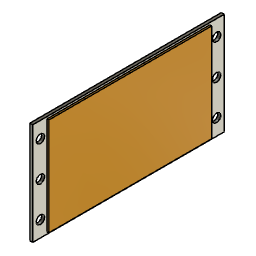
Reflektor v12 (Autodesk Fusion 360 archive; units mm, degrees)
design "LED"
Autodesk Fusion 360 part; units mm, degrees
sketch "Sketch1" plane through (0, 0, 0) normal (1, 0, 0) x (0, 1, 0) in component "Led"
  line L0 (47, 25) -> (-47, 25)
  line L1 (-47, 25) -> (-47, -25)
  line L2 (-47, -25) -> (47, -25)
  line L3 (47, -25) -> (47, 25)
  line L4 (47, 25) -> (-47, -25) construction
  line L5 (-47, 25) -> (47, -25) construction
  line L6 (40, -24) -> (-40, -24)
  line L7 (-40, -24) -> (-40, 24)
  line L8 (-40, 24) -> (40, 24)
  line L9 (40, 24) -> (40, -24)
  line L10 (40, -24) -> (-40, 24) construction
  line L11 (-40, -24) -> (40, 24) construction
  circle A0 centre (43.25, 0) radius 2.05
  line L12 (43.25, 0) -> (43.25, 17.2) construction
  line L13 (43.25, 0) -> (43.25, -17.2) construction
  circle A1 centre (43.25, 17.2) radius 2.05
  circle A2 centre (43.25, -17.2) radius 2.05
  line L14 (0, 25) -> (0, -25) construction
  circle A3 centre (-43.25, 17.2) radius 2.05
  circle A4 centre (-43.25, 0) radius 2.05
  circle A5 centre (-43.25, -17.2) radius 2.05
  line L15 (39.5, 24) -> (-39.5, 24) construction
  line L16 (-39.5, 24) -> (-39.5, -24) construction
  line L17 (-39.5, -24) -> (39.5, -24) construction
  line L18 (39.5, -24) -> (39.5, 24) construction
  line L19 (39.5, 24) -> (-39.5, -24) construction
  line L20 (-39.5, 24) -> (39.5, -24) construction
  line L21 (39.5, 0) -> (47, 0) construction
  dimension "d9" = 94
  dimension "d10" = 50
  dimension "d11" = 80
  dimension "d12" = 48
  dimension "d13" = 4.1
  dimension "d14" = 17.2
  dimension "d15" = 17.2
  dimension "d16" = 4.1
  dimension "d17" = 4.1
  dimension "d24" = 79
  dimension "d25" = 48
  constraint horizontal L0
  constraint perpendicular L0 L1
  constraint parallel L0 L2
  constraint parallel L1 L3
  constraint coincident L4 origin
  constraint coincident L5 origin
  constraint horizontal L6
  constraint perpendicular L6 L7
  constraint parallel L6 L8
  constraint parallel L7 L9
  constraint coincident L10 origin
  constraint coincident L11 origin
  constraint coincident A0.centre L12.start
  constraint perpendicular L2 L13
  constraint coincident L12.end A1.centre
  constraint coincident L13.end A2.centre
  constraint midpoint L0 L14.start
  constraint midpoint L2 L14.end
  constraint symmetric A0 L14 A4
  constraint symmetric A1 L14 A3
  constraint symmetric A2 L14 A5
  constraint horizontal L15
  constraint perpendicular L15 L16
  constraint parallel L15 L17
  constraint parallel L16 L18
  constraint coincident L19 origin
  constraint coincident L20 origin
  constraint midpoint L18 L21.start
  constraint midpoint L3 L21.end
  constraint midpoint A0.centre L21
  constraint parallel L12 L13
  measures "d9" distance of L1.end L2.end
  measures "d10" distance of L0.end L1.end
  measures "d11" distance of L7.end L8.end
  measures "d12" distance of L6.end L7.end
  measures "d13" diameter of A0
  measures "d14" distance of A0.centre L12.end
  measures "d15" distance of A0.centre L13.end
  measures "d16" diameter of A1
  measures "d17" diameter of A2
  measures "d24" distance of L16.end L17.end
  measures "d25" distance of L15.end L16.end
extrude "Extrude1" add sketch "Sketch1" along normal blind 1.4 contours L0 L1 L2 L3 | L6 L7 L8 L9 in component "Led"
extrude "Extrude2" add sketch "Sketch1" along normal blind 2.3 contours L6 L7 L8 L9 in component "Led"
component "Led" placed x (1, 0, 0) y (0, 1, 0) z (0, 0, 1) at (1.4097, 0.3286, -4.1948)
equation "Širina = 94 mm"
equation "mala_širina = 80 mm"
equation "višina = 50 mm"
equation "mala_višina = višina - 2 mm"
equation "razdalja_med_luknjami = 17.2 mm"
equation "fi = 4.1 mm"
equation "debelina = 1.4 mm"
equation "velika_debelina = 2.3 mm"
equation "d9 = Širina"
equation "d10 = višina"
equation "d11 = mala_širina"
equation "d12 = mala_višina"
equation "d13 = fi"
equation "d14 = razdalja_med_luknjami"
equation "d15 = razdalja_med_luknjami"
equation "d16 = fi"
equation "d17 = fi"
equation "d18 = debelina"
equation "d20 = velika_debelina"
equation "namišljena_mala_višina = 79 mm"
equation "d24 = namišljena_mala_višina"
equation "d25 = mala_višina"

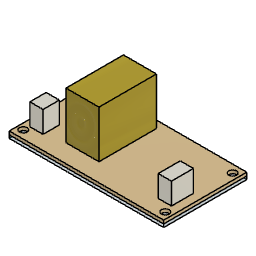
design "Napajalnik 12v 2a"
Autodesk Fusion 360 part; units mm, degrees
sketch "Sketch1" plane through (0, 0, 0) normal (0, 0, 1) x (1, 0, 0)
  line L0 (35.115, -18.89) -> (-35.115, -18.89)
  line L1 (-35.115, -18.89) -> (-35.115, 18.89)
  line L2 (-35.115, 18.89) -> (35.115, 18.89)
  line L3 (35.115, 18.89) -> (35.115, -18.89)
  line L4 (35.115, -18.89) -> (-35.115, 18.89) construction
  line L5 (-35.115, -18.89) -> (35.115, 18.89) construction
  circle A0 centre (-32.37, 15.345) radius 1.745
  circle A1 centre (32.24, 15.345) radius 1.745
  circle A2 centre (-32.37, -15.245) radius 1.745
  circle A3 centre (32.24, -15.245) radius 1.745
  line L6 (31.315, -1.56) -> (25.315, -1.56)
  line L7 (25.315, -1.56) -> (25.315, -11.56)
  line L8 (25.315, -11.56) -> (31.315, -11.56)
  line L9 (31.315, -11.56) -> (31.315, -1.56)
  line L10 (35.115, 15.345) -> (33.985, 15.345) construction
  line L11 (33.985, -15.245) -> (35.115, -15.245) construction
  line L12 (32.24, 18.89) -> (32.24, 17.09) construction
  line L13 (32.24, -16.99) -> (32.24, -18.89) construction
  line L14 (31.315, -11.56) -> (35.115, -11.56) construction
  line L15 (31.315, -11.56) -> (31.315, -18.89) construction
  line L16 (-32.37, -16.99) -> (-32.37, -18.89) construction
  line L17 (-34.115, -15.245) -> (-35.115, -15.245) construction
  line L18 (-32.37, 17.09) -> (-32.37, 18.89) construction
  line L19 (-34.115, 15.345) -> (-35.115, 15.345) construction
  line L20 (-32.115, -5.12) -> (-26.115, -5.12)
  line L21 (-26.115, -5.12) -> (-26.115, -12.52)
  line L22 (-26.115, -12.52) -> (-32.115, -12.52)
  line L23 (-32.115, -12.52) -> (-32.115, -5.12)
  line L24 (-32.115, -12.52) -> (-32.115, -18.89) construction
  line L25 (-32.115, -12.52) -> (-35.115, -12.52) construction
  line L26 (-17.615, 15.55) -> (-2.615, 15.55)
  line L27 (-2.615, 15.55) -> (-2.615, -10.59)
  line L28 (-2.615, -10.59) -> (-17.615, -10.59)
  line L29 (-17.615, -10.59) -> (-17.615, 15.55)
  line L30 (-10.115, -10.59) -> (-10.115, -18.89) construction
  line L31 (-17.615, 15.55) -> (-35.115, 15.345) construction
  dimension "d1" = 70.23
  dimension "d2" = 37.78
  dimension "d3" = 3.49
  dimension "d4" = 3.49
  dimension "d5" = 3.49
  dimension "d6" = 3.49
  dimension "d7" = 6
  dimension "d8" = 10
  dimension "d9" = 1.13
  dimension "d10" = 1.13
  dimension "d11" = 1.8
  dimension "d12" = 1.9
  dimension "d13" = 3.8
  dimension "d14" = 7.33
  dimension "d15" = 1
  dimension "d16" = 1
  dimension "d17" = 6
  dimension "d18" = 7.4
  dimension "d19" = 6.37
  dimension "d20" = 3
  dimension "d21" = 15
  dimension "d22" = 26.14
  dimension "d23" = 8.3
  dimension "d24" = 17.5
  constraint horizontal L0
  constraint perpendicular L0 L1
  constraint parallel L0 L2
  constraint parallel L1 L3
  constraint coincident L4 origin
  constraint coincident L5 origin
  constraint horizontal L6
  constraint vertical L7
  constraint horizontal L8
  constraint vertical L9
  constraint coincident L3 L10.start
  constraint coincident A1 L10.end
  constraint perpendicular L3 L10
  constraint coincident A1.centre L10
  constraint coincident A3 L11.start
  constraint coincident L3 L11.end
  constraint perpendicular L3 L11
  constraint coincident A3.centre L11
  constraint coincident L2 L12.start
  constraint coincident A1 L12.end
  constraint perpendicular L2 L12
  constraint coincident A1.centre L12
  constraint coincident A3 L13.start
  constraint coincident L0 L13.end
  constraint perpendicular L0 L13
  constraint coincident A3.centre L13
  constraint coincident L3 L14.end
  constraint perpendicular L3 L14
  constraint coincident L0 L15.end
  constraint perpendicular L0 L15
  constraint coincident A2 L16.start
  constraint coincident L0 L16.end
  constraint perpendicular L0 L16
  constraint coincident A2.centre L16
  constraint coincident A2 L17.start
  constraint coincident L1 L17.end
  constraint perpendicular L1 L17
  constraint coincident A2.centre L17
  constraint coincident A0 L18.start
  constraint coincident L2 L18.end
  constraint perpendicular L2 L18
  constraint coincident A0 L19.start
  constraint coincident L1 L19.end
  constraint perpendicular L1 L19
  constraint coincident A0.centre L18
  constraint coincident A0.centre L19
  constraint equal L12 L18
  constraint equal L13 L16
  constraint horizontal L20
  constraint vertical L21
  constraint horizontal L22
  constraint vertical L23
  constraint coincident L0 L24.end
  constraint perpendicular L0 L24
  constraint coincident L1 L25.end
  constraint perpendicular L1 L25
  constraint horizontal L26
  constraint vertical L27
  constraint horizontal L28
  constraint vertical L29
  constraint midpoint L28 L30.start
  constraint coincident L0 L30.end
  constraint perpendicular L0 L30
  measures "d1" distance of L1.end L2.end
  measures "d2" distance of L0.end L1.end
  measures "d3" diameter of A0
  measures "d4" diameter of A1
  measures "d5" diameter of A2
  measures "d6" diameter of A3
  measures "d7" distance of L6.start L6.end
  measures "d8" distance of L6.start L8.end
  measures "d9" distance of L10.start L10.end
  measures "d10" distance of L11.start L11.end
  measures "d11" distance of L12.start L12.end
  measures "d12" distance of L13.start L13.end
  measures "d13" distance of L8.end L14.end
  measures "d14" distance of L8.end L15.end
  measures "d15" distance of L19.start L19.end
  measures "d16" distance of L17.start L17.end
  measures "d17" distance of L20.start L20.end
  measures "d18" distance of L20.start L22.end
  measures "d19" distance of L22.end L24.end
  measures "d20" distance of L22.end L25.end
  measures "d21" distance of L26.start L26.end
  measures "d22" distance of L26.start L28.end
  measures "d23" distance of L30.start L30.end
  measures "d24" horizontal distance of L19.end L26.start
extrude "Extrude1" add sketch "Sketch1" against normal blind 1.5 contours L0 L1 L2 L3 | L6 L7 L8 L9 | L20 L21 L22 L23 | L26 L27 L28 L29 makes body 1
extrude "Extrude2" add sketch "Sketch1" along normal blind 21.5 separate body contours L26 L27 L28 L29 makes body 2
extrude "Extrude3" add sketch "Sketch1" along normal blind 9.8 separate body contours L6 L7 L8 L9 | L20 L21 L22 L23 makes body 3 at (31.315, -8.2267, 3.2667) makes body 4 at (-26.115, -7.5867, 6.5333)
ref_plane "WorkPlane1" through (0, 0, -2.9) normal (0, 0, -1) x (-1, 0, 0)
sketch "Sketch2" plane through (0, 0, -2.9) normal (0, 0, -1) x (1, 0, 0)
  line L0 (-35.115, 18.89) -> (35.115, 18.89)
  line L1 (35.115, 18.89) -> (35.115, -18.89)
  line L2 (35.115, -18.89) -> (-35.115, -18.89)
  line L3 (-35.115, -18.89) -> (-35.115, 18.89)
  point P0 (-35.115, 18.89)
  point P1 (35.115, -18.89)
  constraint horizontal L0
  constraint vertical L1
  constraint horizontal L2
  constraint vertical L3
  constraint coincident P0 L0.start
  constraint coincident P1 L1.end
extrude "Extrude4" add sketch "Sketch2" against normal up to surface (1.4 mm away) separate body makes body 5
equation "d1 = 70.13 mm + 0.1 mm"
equation "d27 = 23 mm - 1.5 mm"
equation "d29 = 11.3 mm - 1.5 mm"

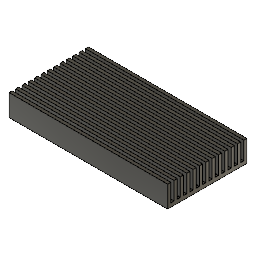
design "Hladilnik"
Autodesk Fusion 360 part; units mm, degrees
sketch "Sketch1" plane through (0, 0, 0) normal (0, 0, 1) x (1, 0, 0)
  line L0 (40, 20) -> (-40, 20)
  line L1 (-40, 20) -> (-40, -20)
  line L2 (-40, -20) -> (40, -20)
  line L3 (40, -20) -> (40, 20)
  line L4 (40, 20) -> (-40, -20) construction
  line L5 (-40, 20) -> (40, -20) construction
  dimension "d4" = 80
  dimension "d5" = 40
  constraint horizontal L0
  constraint perpendicular L0 L1
  constraint parallel L0 L2
  constraint parallel L1 L3
  constraint coincident L4 origin
  constraint coincident L5 origin
  measures "d4" distance of L1.end L2.end
  measures "d5" distance of L0.end L1.end
extrude "Extrude1" add sketch "Sketch1" along normal blind 11
sketch "Sketch2" plane through (-40, 0, 0) normal (-1, 0, 0) x (0, -1, 0)
  line L0 (-20, 0) -> (20, 0)
  line L1 (20, 0) -> (20, 11)
  line L2 (20, 11) -> (-20, 11)
  line L3 (-20, 11) -> (-20, 0)
  line L4 (-20, 11) -> (-18.4, 11)
  line L5 (-18.4, 11) -> (-18.4, 2)
  line L6 (-18.4, 2) -> (-16.8, 2)
  line L7 (-16.8, 2) -> (-16.8, 11)
  line L8 (-16.8, 11) -> (-15.2, 11)
  line L9 (-15.2, 11) -> (-15.2, 2)
  line L10 (-15.2, 2) -> (-13.6, 2)
  line L11 (-13.6, 2) -> (-13.6, 11)
  line L12 (-13.6, 11) -> (-12, 11)
  line L13 (-12, 11) -> (-12, 2)
  line L14 (-12, 2) -> (-10.4, 2)
  line L15 (-10.4, 2) -> (-10.4, 11)
  line L16 (-10.4, 11) -> (-8.8, 11)
  line L17 (-8.8, 11) -> (-8.8, 2)
  line L18 (-8.8, 2) -> (-7.2, 2)
  line L19 (-7.2, 2) -> (-7.2, 11)
  line L20 (-7.2, 11) -> (-5.6, 11)
  line L21 (-5.6, 11) -> (-5.6, 2)
  line L22 (-5.6, 2) -> (-4, 2)
  line L23 (-4, 2) -> (-4, 11)
  line L24 (-4, 11) -> (-2.4, 11)
  line L25 (-2.4, 11) -> (-2.4, 2)
  line L26 (-2.4, 2) -> (-0.8, 2)
  line L27 (-0.8, 2) -> (-0.8, 11)
  line L28 (-0.8, 11) -> (0.8, 11)
  line L29 (0.8, 11) -> (0.8, 2)
  line L30 (0.8, 2) -> (2.4, 2)
  line L31 (2.4, 2) -> (2.4, 11)
  line L32 (2.4, 11) -> (4, 11)
  line L33 (4, 11) -> (4, 2)
  line L34 (4, 2) -> (5.6, 2)
  line L35 (5.6, 2) -> (5.6, 11)
  line L36 (5.6, 11) -> (7.2, 11)
  line L37 (7.2, 11) -> (7.2, 2)
  line L38 (7.2, 2) -> (8.8, 2)
  line L39 (8.8, 2) -> (8.8, 11)
  line L40 (8.8, 11) -> (10.4, 11)
  line L41 (10.4, 11) -> (10.4, 2)
  line L42 (10.4, 2) -> (12, 2)
  line L43 (12, 2) -> (12, 11)
  line L44 (12, 11) -> (13.6, 11)
  line L45 (13.6, 11) -> (13.6, 2)
  line L46 (13.6, 2) -> (15.2, 2)
  line L47 (15.2, 2) -> (15.2, 11)
  line L48 (15.2, 11) -> (16.8, 11)
  line L49 (16.8, 11) -> (16.8, 2)
  line L50 (16.8, 2) -> (18.4, 2)
  line L51 (18.4, 2) -> (18.4, 11)
  line L52 (18.4, 11) -> (20, 11)
  dimension "d9" = 1.6
  dimension "d11" = 9
  dimension "d12" = 1.6
  dimension "d13" = 9
  dimension "d14" = 1.6
  dimension "d15" = 9
  dimension "d16" = 1.6
  dimension "d17" = 9
  dimension "d18" = 1.6
  dimension "d19" = 9
  dimension "d20" = 1.6
  dimension "d21" = 9
  dimension "d22" = 1.6
  dimension "d23" = 9
  dimension "d24" = 1.6
  dimension "d25" = 9
  dimension "d26" = 1.6
  dimension "d27" = 9
  dimension "d28" = 1.6
  dimension "d29" = 9
  dimension "d30" = 1.6
  dimension "d31" = 9
  dimension "d32" = 1.6
  dimension "d33" = 9
  dimension "d34" = 1.6
  dimension "d35" = 9
  dimension "d36" = 1.6
  dimension "d37" = 9
  dimension "d38" = 1.6
  dimension "d39" = 9
  dimension "d40" = 1.6
  dimension "d41" = 9
  dimension "d42" = 1.6
  dimension "d43" = 9
  dimension "d44" = 1.6
  dimension "d45" = 9
  dimension "d46" = 1.6
  dimension "d47" = 9
  dimension "d48" = 1.6
  dimension "d49" = 9
  dimension "d50" = 1.6
  dimension "d51" = 9
  dimension "d52" = 1.6
  dimension "d53" = 9
  dimension "d54" = 1.6
  dimension "d55" = 9
  dimension "d56" = 1.6
  dimension "d57" = 9
  dimension "d58" = 1.6
  constraint coincident L2.end L3.start
  constraint perpendicular L3 L4
  constraint perpendicular L0 L5
  constraint perpendicular L5 L6
  constraint perpendicular L2 L7
  constraint coincident L2 L8.end
  constraint perpendicular L2 L9
  constraint perpendicular L9 L10
  constraint perpendicular L2 L11
  constraint perpendicular L11 L12
  constraint perpendicular L2 L13
  constraint perpendicular L11 L14
  constraint perpendicular L2 L15
  constraint perpendicular L15 L16
  constraint perpendicular L2 L17
  constraint perpendicular L15 L18
  constraint perpendicular L2 L19
  constraint perpendicular L19 L20
  constraint perpendicular L2 L21
  constraint perpendicular L21 L22
  constraint perpendicular L2 L23
  constraint perpendicular L23 L24
  constraint perpendicular L2 L25
  constraint perpendicular L25 L26
  constraint perpendicular L2 L27
  constraint perpendicular L27 L28
  constraint perpendicular L2 L29
  constraint perpendicular L29 L30
  constraint perpendicular L2 L31
  constraint perpendicular L31 L32
  constraint perpendicular L32 L33
  constraint perpendicular L33 L34
  constraint perpendicular L2 L35
  constraint perpendicular L35 L36
  constraint perpendicular L36 L37
  constraint perpendicular L37 L38
  constraint perpendicular L2 L39
  constraint perpendicular L39 L40
  constraint perpendicular L40 L41
  constraint perpendicular L41 L42
  constraint perpendicular L2 L43
  constraint perpendicular L41 L44
  constraint perpendicular L44 L45
  constraint perpendicular L45 L46
  constraint perpendicular L2 L47
  constraint perpendicular L47 L48
  constraint perpendicular L48 L49
  constraint perpendicular L47 L50
  constraint perpendicular L2 L51
  constraint perpendicular L1 L52
  measures "d9" distance of L2.end L4.end
  measures "d11" distance of L4.end L5.end
  measures "d12" distance of L5.end L6.end
  measures "d13" distance of L6.end L7.end
  measures "d14" distance of L7.end L8.end
  measures "d15" distance of L8.end L9.end
  measures "d16" distance of L9.end L10.end
  measures "d17" distance of L10.end L11.end
  measures "d18" distance of L11.end L12.end
  measures "d19" distance of L12.end L13.end
  measures "d20" distance of L13.end L14.end
  measures "d21" distance of L14.end L15.end
  measures "d22" distance of L15.end L16.end
  measures "d23" distance of L16.end L17.end
  measures "d24" distance of L17.end L18.end
  measures "d25" distance of L18.end L19.end
  measures "d26" distance of L19.end L20.end
  measures "d27" distance of L20.end L21.end
  measures "d28" distance of L21.end L22.end
  measures "d29" distance of L22.end L23.end
  measures "d30" distance of L23.end L24.end
  measures "d31" distance of L24.end L25.end
  measures "d32" distance of L25.end L26.end
  measures "d33" distance of L26.end L27.end
  measures "d34" distance of L27.end L28.end
  measures "d35" distance of L28.end L29.end
  measures "d36" distance of L29.end L30.end
  measures "d37" distance of L30.end L31.end
  measures "d38" distance of L31.end L32.end
  measures "d39" distance of L32.end L33.end
  measures "d40" distance of L33.end L34.end
  measures "d41" distance of L34.end L35.end
  measures "d42" distance of L35.end L36.end
  measures "d43" distance of L36.end L37.end
  measures "d44" distance of L37.end L38.end
  measures "d45" distance of L38.end L39.end
  measures "d46" distance of L39.end L40.end
  measures "d47" distance of L40.end L41.end
  measures "d48" distance of L41.end L42.end
  measures "d49" distance of L42.end L43.end
  measures "d50" distance of L43.end L44.end
  measures "d51" distance of L44.end L45.end
  measures "d52" distance of L45.end L46.end
  measures "d53" distance of L46.end L47.end
  measures "d54" distance of L47.end L48.end
  measures "d55" distance of L48.end L49.end
  measures "d56" distance of L49.end L50.end
  measures "d57" distance of L50.end L51.end
  measures "d58" distance of L51.end L1.end
extrude "Extrude2" cut sketch "Sketch2" against normal up to surface (80 mm away) contours L2 L5 L6 L7 | L2 L49 L50 L51 | L2 L9 L10 L11 | L2 L45 L46 L47 | L2 L13 L14 L15 | L2 L41 L42 L43 | L2 L17 L18 L19 | L2 L37 L38 L39 | L2 L21 L22 L23 | L2 L33 L34 L35 | L2 L25 L26 L27 | L2 L29 L30 L31
equation "x = 80 mm"
equation "y = 40 mm"
equation "z = 11 mm"
equation "d4 = x"
equation "d5 = y"
equation "d6 = z"
equation "u = y / ( 13 * 2 - 1 )"
equation "d9 = u"
equation "v = 9 mm"
equation "d11 = v"
equation "d12 = u"
equation "d13 = v"
equation "d14 = u"
equation "d15 = v"
equation "d16 = u"
equation "d17 = v"
equation "d18 = u"
equation "d19 = v"
equation "d20 = u"
equation "d21 = v"
equation "d22 = u"
equation "d23 = v"
equation "d24 = u"
equation "d25 = v"
equation "d26 = u"
equation "d27 = v"
equation "d28 = u"
equation "d29 = v"
equation "d30 = u"
equation "d31 = v"
equation "d32 = u"
equation "d33 = v"
equation "d34 = u"
equation "d35 = v"
equation "d37 = v"
equation "d38 = u"
equation "d39 = v"
equation "d40 = u"
equation "d41 = v"
equation "d42 = u"
equation "d43 = v"
equation "d44 = u"
equation "d45 = v"
equation "d46 = u"
equation "d47 = v"
equation "d48 = u"
equation "d49 = v"
equation "d50 = u"
equation "d51 = v"
equation "d52 = u"
equation "d53 = v"
equation "d54 = u"
equation "d55 = v"
equation "d56 = u"
equation "d57 = v"
equation "d58 = u"

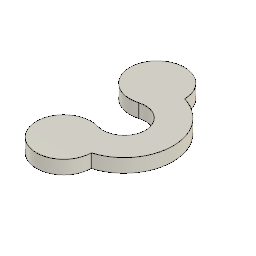
design "M3 click"
Autodesk Fusion 360 part; units mm, degrees
sketch "Sketch1" plane through (0, 0, 0) normal (0, 0, 1) x (1, 0, 0)
  circle A0 centre (0, 0) radius 1.55
  circle A1 centre (-1, 3.4062) radius 2
  circle A2 centre (-1, -3.4062) radius 2
  line L0 (-1, 3.4062) -> (-1, -3.4062) construction
  circle A3 centre (0, 0) radius 3.55
  line L1 (0, 0) -> (-1, 0) construction
  dimension "d1" = 3.1
  dimension "d2" = 4
  dimension "d4" = 1
  dimension "d7" = 2
  constraint coincident A0.centre A3.centre
  constraint equal A1 A2
  constraint tangent A0 A1
  constraint tangent A0 A2
  constraint coincident A1.centre L0.start
  constraint coincident A2.centre L0.end
  constraint vertical L0
  constraint horizontal L1
  constraint coincident L0 L1.end
  measures "d1" diameter of A0
  measures "d2" diameter of A1
  measures "d4" distance of A0.centre L1.end
extrude "Extrude1" add sketch "Sketch1" along normal blind 1 contours A0 A1 A2 A3 | A1 A3 | A2 A3 | A1 A3 | A2 A3 picked at (1.3407, -2.0598)
